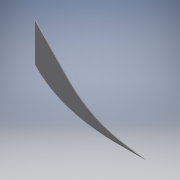
# Autodesk Inventor part: splitter
Saved by Autodesk Inventor 2018 (Build 220112000, 112)
## iProperties
Created: 2018-05-16
Part Number: splitter
Material: 一般
Document SubType Name: Modeling
Designer: ku_sk
Density: 1 g/cm^3
Appearance: 既定
Author: ku_sk
Autodesk Inventor part; units mm, degrees
ref_plane "YZ Plane" through (0, 0, 0) normal (1, 0, 0) x (0, 1, 0)
ref_plane "XZ Plane" through (0, 0, 0) normal (0, 1, 0) x (-1, 0, 0)
ref_plane "XY Plane" through (0, 0, 0) normal (0, 0, 1) x (1, 0, 0)
sketch "スケッチ1" plane through (0, 0, 0) normal (0, 1, 0) x (-1, 0, 0)
  line L0 (101.7324, -28.9004) -> (451.7324, -28.9004)
  line L1 (451.7324, -28.9004) -> (451.7324, 67.6956)
  arc A0 (451.7324, 67.6956) -> (328.1926, 37.3714) centre (451.7324, -199.1148) ccw
  arc A1 (101.7324, -28.9004) -> (328.1926, 37.3714) centre (48.6916, 572.4068) ccw
  dimension "d1" = 350
  dimension "d2" = 603.642
  constraints: 4 end point, 4 point on circle, 2 centre point, 1 line through centre, 1 perpendicular
  measures "d1" distance of L0.start L0.end
  measures "d2" radius of A1
extrude "押し出し1" add sketch "スケッチ1" along normal blind 70
sketch "スケッチ2" plane through (-101.7324, 0, -28.9004) normal (0, 0, -1) x (-1, 0, 0)
  arc A0 (68.7528, 0) -> (350, 70) centre (68.7528, 600) ccw
  line L0 (350, 0) -> (0, 0) projected
  line L1 (350, 0) -> (350, 70) projected
  line L2 (0, 0) -> (0, 70) projected
  point P0 (-101.7324, 0)
  dimension "d9" = 600
  constraints: 2 point on circle, 1 centre point, 1 coincident, 1 point on line, 1 tangent
  measures "d9" radius of A0
extrude "押し出し2" cut sketch "スケッチ2" against normal through all
shell "シェル1" thickness 2 removed faces 4 at (-334.0598, 39.1147, 40.3449) at (-359.2071, 70, 10.3289) at (-150.6861, 46.6667, -22.5561) at (-325.356, 65.1801, -28.9004)
